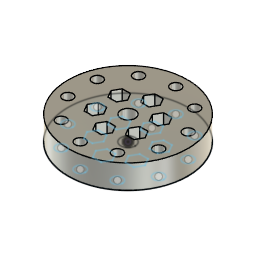
Reakcion_Wheel v4 (Autodesk Fusion 360 design; units mm, degrees)
Autodesk Fusion 360 part; units mm, degrees
sketch "Sketch1" plane through (0, 0, 0) normal (0, 0, 1) x (1, 0, 0)
  circle A0 centre (0, 0) radius 50
  circle A1 centre (0, 40) radius 4.25
  circle A2 centre (-23.5114, 32.3607) radius 4.25
  circle A3 centre (-38.0423, 12.3607) radius 4.25
  circle A4 centre (-38.0423, -12.3607) radius 4.25
  circle A5 centre (-23.5114, -32.3607) radius 4.25
  circle A6 centre (0, -40) radius 4.25
  circle A7 centre (23.5114, -32.3607) radius 4.25
  circle A8 centre (38.0423, -12.3607) radius 4.25
  circle A9 centre (38.0423, 12.3607) radius 4.25
  circle A10 centre (23.5114, 32.3607) radius 4.25
  line L0 (-3.4339, 13.9827) -> (3.4942, 14.0175)
  line L1 (3.4942, 14.0175) -> (6.9281, 20.0348)
  line L2 (6.9281, 20.0348) -> (3.4339, 26.0173)
  line L3 (3.4339, 26.0173) -> (-3.4942, 25.9825)
  line L4 (-3.4942, 25.9825) -> (-6.9281, 19.9652)
  line L5 (-6.9281, 19.9652) -> (-3.4339, 13.9827)
  line L6 (-20.7544, 3.9827) -> (-13.8263, 4.0175)
  line L7 (-13.8263, 4.0175) -> (-10.3924, 10.0348)
  line L8 (-10.3924, 10.0348) -> (-13.8866, 16.0173)
  line L9 (-13.8866, 16.0173) -> (-20.8147, 15.9825)
  line L10 (-24.2486, 9.9652) -> (-20.7544, 3.9827)
  line L11 (-20.8147, 15.9825) -> (-24.2486, 9.9652)
  line L12 (-13.8263, -15.9825) -> (-10.3924, -9.9652)
  line L13 (-10.3924, -9.9652) -> (-13.8866, -3.9827)
  line L14 (-13.8866, -3.9827) -> (-20.8147, -4.0175)
  line L15 (-20.8147, -4.0175) -> (-24.2486, -10.0348)
  line L16 (-20.7544, -16.0173) -> (-13.8263, -15.9825)
  line L17 (-24.2486, -10.0348) -> (-20.7544, -16.0173)
  line L18 (6.9281, -19.9652) -> (3.4339, -13.9827)
  line L19 (3.4339, -13.9827) -> (-3.4942, -14.0175)
  line L20 (-3.4942, -14.0175) -> (-6.9281, -20.0348)
  line L21 (-6.9281, -20.0348) -> (-3.4339, -26.0173)
  line L22 (3.4942, -25.9825) -> (6.9281, -19.9652)
  line L23 (-3.4339, -26.0173) -> (3.4942, -25.9825)
  line L24 (20.7544, -3.9827) -> (13.8263, -4.0175)
  line L25 (13.8263, -4.0175) -> (10.3924, -10.0348)
  line L26 (10.3924, -10.0348) -> (13.8866, -16.0173)
  line L27 (13.8866, -16.0173) -> (20.8147, -15.9825)
  line L28 (24.2486, -9.9652) -> (20.7544, -3.9827)
  line L29 (20.8147, -15.9825) -> (24.2486, -9.9652)
  line L30 (13.8263, 15.9825) -> (10.3924, 9.9652)
  line L31 (10.3924, 9.9652) -> (13.8866, 3.9827)
  line L32 (13.8866, 3.9827) -> (20.8147, 4.0175)
  line L33 (20.8147, 4.0175) -> (24.2486, 10.0348)
  line L34 (20.7544, 16.0173) -> (13.8263, 15.9825)
  line L35 (24.2486, 10.0348) -> (20.7544, 16.0173)
  circle A11 centre (0, 0) radius 6
  point P0 (0, 20)
  dimension "d3" = 100
  dimension "d4" = 8.5
  dimension "d5" = 40
  dimension "d7" = 360
  dimension "d9" = 6
  dimension "d10" = 20
  dimension "d12" = 360
  dimension "d16" = 12
  constraint coincident A0.centre A11.centre
  constraint concentric A0 A11
  measures "d3" diameter of A0
  measures "d4" diameter of A1
  measures "d5" distance of A0.centre A1.centre
  measures "d9" distance of P0 L5
  measures "d10" distance of A0.centre P0
  measures "d16" diameter of A11
extrude "Extrude1" add sketch "Sketch1" along normal blind 20 contours A0 | A11 makes body 1
copy_body "Body->Comp1" bodies 1 removing the originals makes body 2 in component "Component"
extrude "Extrude1'" cut sketch "Sketch1" along normal blind 21.019 contours A11 bodies 2 in component "Component"
component "Component" placed x (1, 0, 0) y (0, 1, 0) z (0, 0, 1) at (0, 0, 0)
equation "Reaktion_Durchmesser = 120 mm"
equation "M8_Durchmesser = 8.5 mm"
equation "d4 = M8_Durchmesser"
equation "Plygon_D = 6 mm"
equation "wheel_hohe = 20 mm"
equation "d14 = wheel_hohe"
